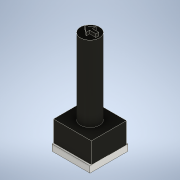
# Autodesk Inventor part: f18base
Saved by Autodesk Inventor 2021 (Build 250183000, 183)
## iProperties
Created: 2023-12-10
Part Number: f18base
Material: Generic
Document SubType Name: Modeling
Designer: assman
Density: 1 g/cm^3
Appearance: Default
Author: assman
Autodesk Inventor part; units mm, degrees
ref_plane "YZ Plane" through (0, 0, 0) normal (1, 0, 0) x (0, 1, 0)
ref_plane "XZ Plane" through (0, 0, 0) normal (0, 1, 0) x (-1, 0, 0)
ref_plane "XY Plane" through (0, 0, 0) normal (0, 0, 1) x (1, 0, 0)
sketch "Sketch1" plane through (0, 0, 0) normal (0, 1, 0) x (-1, 0, 0)
  line L0 (60, 55.5) -> (-60, 55.5) construction
  line L1 (-60, 55.5) -> (-60, -55.5) construction
  line L2 (-60, -55.5) -> (60, -55.5) construction
  line L3 (60, -55.5) -> (60, 55.5) construction
  line L4 (60, 55.5) -> (-60, -55.5) construction
  line L5 (-60, 55.5) -> (60, -55.5) construction
  line L6 (30.05, 30.05) -> (-30.05, 30.05) construction
  line L7 (-30.05, 30.05) -> (-30.05, -30.05) construction
  line L8 (-30.05, -30.05) -> (30.05, -30.05) construction
  line L9 (30.05, -30.05) -> (30.05, 30.05) construction
  line L10 (30.05, 30.05) -> (-30.05, -30.05) construction
  line L11 (-30.05, 30.05) -> (30.05, -30.05) construction
  circle A0 centre (30.05, 30.05) radius 2
  circle A1 centre (30.05, -30.05) radius 2
  circle A2 centre (-30.05, 30.05) radius 2
  circle A3 centre (-30.05, -30.05) radius 2
  line L12 (60, 60) -> (-60, 60)
  line L13 (-60, 60) -> (-60, -60)
  line L14 (-60, -60) -> (60, -60)
  line L15 (60, -60) -> (60, 60)
  line L16 (60, 60) -> (-60, -60) construction
  line L17 (-60, 60) -> (60, -60) construction
  point P0 (0, 0)
  point P1 (0, 0)
  point P2 (0, 0)
  dimension "d0" = 120
  dimension "d1" = 111
  dimension "d2" = 60.1
  dimension "d3" = 60.1
  dimension "d4" = 4
  dimension "d5" = 4
  dimension "d6" = 4
  dimension "d7" = 4
  dimension "d8" = 120
  dimension "d9" = 120
  constraints: 36 end point, 8 midpoint, 6 parallel, 4 centre point, 3 horizontal, 3 perpendicular, 2 coincident
  measures "d0" distance of L2.end L1.end
  measures "d1" distance of L1.end L0.end
  measures "d2" distance of L8.end L7.end
  measures "d3" distance of L7.end L6.end
  measures "d4" diameter of A0
  measures "d5" diameter of A1
  measures "d6" diameter of A2
  measures "d7" diameter of A3
  measures "d8" distance of L14.end L13.end
  measures "d9" distance of L13.end L12.end
extrude "Extrusion1" add sketch "Sketch1" against normal blind 20
sketch "Sketch2" plane through (0, 0, 0) normal (0, 1, 0) x (1, 0, 0)
  line L0 (-60, -55.5) -> (60, -55.5)
  line L1 (60, -55.5) -> (60, 55.5)
  line L2 (60, 55.5) -> (-60, 55.5)
  line L3 (-60, 55.5) -> (-60, -55.5)
  line L4 (-60, -55.5) -> (60, 55.5) construction
  line L5 (60, -55.5) -> (-60, 55.5) construction
  point P0 (0, 0)
  dimension "d12" = 120
  dimension "d13" = 111
  constraints: 12 end point, 2 midpoint, 2 parallel, 1 horizontal, 1 perpendicular
  measures "d12" distance of L2.end L1.end
  measures "d13" distance of L1.end L0.end
extrude "Extrusion2" add sketch "Sketch2" along normal blind 66 separate body
sketch "Sketch3" plane through (0, 66, 0) normal (0, 1, 0) x (1, 0, 0)
  circle A0 centre (0, 0) radius 30
  dimension "d16" = 60
  constraints: 1 centre point, 1 coincident
  measures "d16" diameter of A0
extrude "Extrusion3" add sketch "Sketch3" along normal blind 239 bodies 2
sketch "Sketch4" plane through (0, 305, 0) normal (0, 1, 0) x (1, 0, 0)
  line L0 (3.3181, 4.3136) -> (23.2268, 4.3136)
  line L1 (23.2268, 4.3136) -> (23.2268, -4.3136)
  line L2 (23.2268, -4.3136) -> (3.3181, -4.3136)
  line L3 (3.3181, -4.3136) -> (3.3181, 4.3136)
  line L4 (3.3181, 4.3136) -> (23.2268, -4.3136) construction
  line L5 (23.2268, 4.3136) -> (3.3181, -4.3136) construction
  line L6 (3.3181, 4.3136) -> (3.3181, 16.3136)
  line L7 (3.3181, 16.3136) -> (-16.0929, 0)
  line L8 (-16.0929, 0) -> (3.3181, -15.5951)
  line L9 (3.3181, -15.5951) -> (3.3181, -3.5951)
  point P0 (0, 0)
  point P1 (13.2725, 0)
  dimension "d19" = 12
  dimension "d20" = 12
  constraints: 20 end point, 2 midpoint, 2 parallel, 2 point on line, 1 horizontal, 1 perpendicular, 1 vertical
  measures "d19" distance of L0.start L6.end
  measures "d20" distance of L8.end L9.end
extrude "Extrusion4" add sketch "Sketch4" along normal blind 10 bodies 2
body "Solid1"
body "Solid2"
